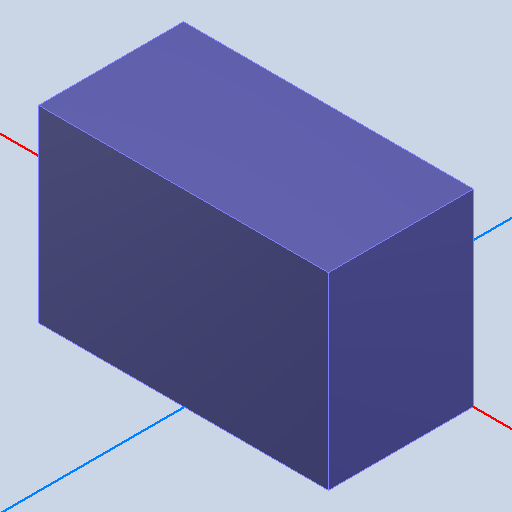
# Autodesk Inventor part: C0805K
Saved by Autodesk Inventor 2022 (Build 260153000, 153)
## iProperties
Created: 2022-02-26
Part Number: C0805K
Material: Типовые
Document SubType Name: Modeling
Designer: Petrov Ivan
Density: 1 g/cm^3
Appearance: C0805K, C0805K
Author: Petrov Ivan
Autodesk Inventor part; units mm, degrees
ref_plane "YZ Plane" through (0, 0, 0) normal (1, 0, 0) x (0, 1, 0)
ref_plane "XZ Plane" through (0, 0, 0) normal (0, 1, 0) x (-1, 0, 0)
ref_plane "XY Plane" through (0, 0, 0) normal (0, 0, 1) x (1, 0, 0)
sketch "C0805K, C0805K_1" plane through (0, 0, 0) normal (0, 0, 1) x (1, 0, 0)
  line L0 (-1, 0.6508) -> (1, 0.6508)
  line L1 (1, 0.6508) -> (1, -0.65)
  line L2 (1, -0.65) -> (-1, -0.65)
  line L3 (-1, -0.65) -> (-1, 0.6508)
  constraints: 8 end point
extrude "Выдавливание1" add sketch "C0805K, C0805K_1" along normal blind 1
